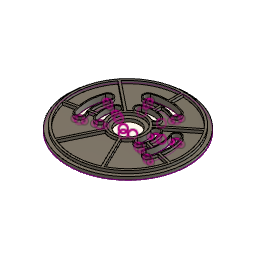
BoschRouterInsert (Autodesk Fusion 360 design; units mm, degrees)
Autodesk Fusion 360 part; units mm, degrees
sketch "Sketch1" plane through (0, 0, 0) normal (0, 1, 0) x (1, 0, 0)
  circle A0 centre (0, 0) radius 48.6
  circle A1 centre (0, 0) radius 9.35
  circle A2 centre (6.6396, 16.0293) radius 3
  circle A3 centre (-6.6396, 16.0293) radius 3
  arc A4 (7.7876, 18.8009) -> (-7.7876, 18.8009) centre (0, 0) ccw
  arc A5 (5.4915, 13.2577) -> (-5.4915, 13.2577) centre (0, 0) ccw
  line L0 (0, 55) -> (0, -55) construction
  circle A6 centre (-6.6396, 16.0293) radius 3.9
  circle A7 centre (6.6396, 16.0293) radius 3.9
  line L1 (0, 0) -> (25.3139, 61.1131) construction
  circle A8 centre (11.5379, 27.855) radius 3
  circle A9 centre (11.5379, 27.855) radius 3.9
  circle A10 centre (-11.5379, 27.855) radius 3
  circle A11 centre (-11.5379, 27.855) radius 3.9
  arc A12 (13.0304, 31.4581) -> (-13.0351, 31.4562) centre (0.0002, -3.0538) ccw
  arc A13 (10.0454, 24.2518) -> (-10.0454, 24.2518) centre (0, 0) ccw
  arc A14 (10.3899, 25.0833) -> (-10.3899, 25.0833) centre (0, 0) ccw
  arc A15 (12.686, 30.6266) -> (-12.6872, 30.6261) centre (0.0001, -3.8821) ccw
  arc A16 (8.132, 19.6324) -> (-8.132, 19.6324) centre (0, 0) ccw
  arc A17 (5.1471, 12.4262) -> (-5.1471, 12.4262) centre (0, 0) ccw
  dimension "d1" = 97.2
  dimension "d7" = 18.7
  dimension "d27" = 6
  dimension "d30" = 5
  dimension "d39" = 0.9
  dimension "d43" = 22.5
  dimension "d44" = 6
  dimension "d46" = 0.9
  dimension "d48" = 0.9
  dimension "d49" = 0.9
  dimension "d50" = 5
  constraint coincident A0.centre A1.centre
  constraint concentric A0 A1
  constraint coincident A3 A4.end
  constraint coincident A2 A4.start
  constraint coincident A3 A5.end
  constraint coincident A2 A5.start
  constraint tangent A2 A5
  constraint tangent A2 A4
  constraint tangent A3 A5
  constraint tangent A3 A4
  constraint vertical L0
  constraint symmetric A2 A3 L0
  constraint concentric A3 A6
  constraint concentric A2 A7
  constraint coincident A2.centre L1
  constraint coincident L1 A8.centre
  constraint concentric A8 A9
  constraint concentric A10 A11
  constraint symmetric L0 A8 A10
  constraint coincident A11 A12.end
  constraint coincident L1 A12.start
  constraint coincident A9 A12.start
  constraint coincident A11 A13.end
  constraint coincident L1 A13.start
  constraint coincident A9 A13.start
  constraint coincident A10 A14.end
  constraint coincident A8 A14.start
  constraint coincident L1 A14.start
  constraint coincident A10 A15.end
  constraint coincident A8 A15.start
  constraint coincident L1 A15.start
  constraint coincident A6 A16.end
  constraint coincident A7 A16.start
  constraint coincident L1 A16.start
  constraint coincident A6 A17.end
  constraint coincident L1 A17.start
  constraint coincident A7 A17.start
  measures "d1" diameter of A0
  measures "d7" diameter of A1
  measures "d27" diameter of A2
  measures "d30" distance of A1 A5
  measures "d39" distance of A3 A6
  measures "d43" angle of L0 L1
  measures "d44" diameter of A8
  measures "d46" distance of A8 A9
  measures "d48" distance of A10 A11
  measures "d49" distance of A2 A7
  measures "d50" distance of A13 A16
extrude "Extrude1" add sketch "Sketch1" along normal blind 2.5 contours A0 | A2 | A2 A4 A5 A7 | A2 A4 A5 A7 | A4 A5 A6 A7 | A4 A6 A7 A16 | A5 A6 A7 A17 | A3 A4 A5 A6 | A3 A4 A5 A6 | A3 | A8 A15 | A8 A9 A12 A14 A15 | A8 A15 | A8 A9 A14 A15 | A9 A11 A14 A15 | A9 A11 A13 A14 | A9 A11 A12 A15 | A10 A11 A14 A15 | A10 A11 A12 A14 A15 | A10 A15 | A10 A15
sketch "support_ribs" plane through (0, 2.5, 0) normal (0, 1, 0) x (-1, 0, 0)
  circle A0 centre (0, 0) radius 9.35
  circle A1 centre (0, 0) radius 48.6
  circle A2 centre (0, 0) radius 45.8
  circle A3 centre (0, 0) radius 44
  circle A4 centre (0, 0) radius 12.35
  circle A5 centre (0, 0) radius 14.15
  line L0 (-0.9352, -13.25) -> (0.8648, -13.25)
  line L1 (0.8648, -13.25) -> (0.8648, -44.9)
  line L2 (0.8648, -44.9) -> (-0.9352, -44.9)
  line L3 (-0.9352, -44.9) -> (-0.9352, -13.25)
  line L4 (-0.9352, -13.25) -> (0.8648, -44.9) construction
  line L5 (0.8648, -13.25) -> (-0.9352, -44.9) construction
  point P0 (-0.0352, -29.075)
  point P1 (-0.0352, -29.075)
  dimension "d12" = 91.6
  dimension "d13" = 88
  dimension "d14" = 24.7
  dimension "d15" = 28.3
  dimension "d16" = 29.075
  dimension "d17" = 1.8
  dimension "d18" = 31.65
  constraint coincident A0.centre A1.centre
  constraint concentric A2 A3
  constraint concentric A3 A4
  constraint perpendicular L0 L1
  constraint parallel L0 L2
  constraint parallel L1 L3
  constraint horizontal L0
  constraint coincident L4 P1
  constraint coincident L5 P1
  constraint coincident P1 P0
  measures "d12" diameter of A2
  measures "d13" diameter of A3
  measures "d14" diameter of A4
  measures "d15" diameter of A5
  measures "d16" vertical distance of A0.centre P1
  measures "d17" distance of L1.end L2.end
  measures "d18" distance of L0.end L1.end
extrude "Extrude2" add sketch "support_ribs" along normal blind 2.3 contours A2 | A3 L1 L2 L3 | A5 L0 L1 L3 | A5 L0 L1 L3
extrude "Extrude3" add sketch "support_ribs" along normal blind 2.3 contours A3 A5 L1 L3 picked at (-0.1352, -24.0974)
pattern_circular "C-Pattern1" count 7 over 360 about axis through (0, 1.75, 0) along (0, 1, 0) of "Extrude3"
extrude "Extrude5" add sketch "Sketch1" along normal blind 4.8 contours A2 A4 A5 A7 | A2 A4 A5 A7 | A4 A5 A6 A7 | A4 A6 A7 A16 | A5 A6 A7 A17 | A3 A4 A5 A6 | A3 A4 A5 A6 | A3 | A8 A9 A12 A14 A15 | A8 A9 A14 A15 | A9 A11 A14 A15 | A9 A11 A13 A14 | A9 A11 A12 A15 | A10 A11 A14 A15 | A10 A11 A12 A14 A15
extrude "Extrude4" cut sketch "Sketch1" along normal blind 14.8 contours A2 | A2 A4 A5 A7 | A4 A5 A6 A7 | A3 A4 A5 A6 | A3 | A8 A15 | A8 A15 | A8 A9 A14 A15 | A9 A11 A14 A15 | A10 A11 A14 A15 | A10 A15 | A10 A15 picked at (5.641, 19.3079) picked at (-5.6852, 19.3231)
chamfer "Chamfer1" distance 0.5 angle 45 4 edges at (0, 0, -14.35) (9.4112, 0, -14.8813) (0, 0, -20.35) (-9.4112, 0, -14.8813)
pattern_circular "C-Pattern2" count 3 over 180 about axis through (0, 1.75, 0) along (0, 1, 0) both ways of "Extrude5", "Extrude4", "Chamfer1"
sketch "Sketch3" plane through (0, 0, 0) normal (0, -1, 0) x (1, 0, 0)
  circle A0 centre (0, 0) radius 9.35
  arc A1 (-5.3002, -12.7957) -> (5.3002, -12.7957) centre (0, 0) ccw
  arc A2 (7.9789, -19.2629) -> (5.3002, -12.7957) centre (6.6396, -16.0293) ccw
  arc A3 (-7.9789, -19.2629) -> (7.9789, -19.2629) centre (0, 0) ccw
  arc A4 (-5.3002, -12.7957) -> (-7.9789, -19.2629) centre (-6.6396, -16.0293) ccw
  arc A5 (12.7957, -5.3002) -> (12.7957, 5.3002) centre (0, 0) ccw
  arc A6 (19.2629, 7.9789) -> (12.7957, 5.3002) centre (16.0293, 6.6396) ccw
  arc A7 (19.2629, -7.9789) -> (19.2629, 7.9789) centre (0, 0) ccw
  arc A8 (12.7957, -5.3002) -> (19.2629, -7.9789) centre (16.0293, -6.6396) ccw
  arc A9 (-12.7957, 5.3002) -> (-12.7957, -5.3002) centre (0, 0) ccw
  arc A10 (-19.2629, -7.9789) -> (-12.7957, -5.3002) centre (-16.0293, -6.6396) ccw
  arc A11 (-19.2629, 7.9789) -> (-19.2629, -7.9789) centre (0, 0) ccw
  arc A12 (-12.7957, 5.3002) -> (-19.2629, 7.9789) centre (-16.0293, 6.6396) ccw
  arc A13 (25.0833, -10.3899) -> (25.0833, 10.3899) centre (0, 0) ccw
  arc A14 (30.7168, 12.4379) -> (25.0833, 10.3899) centre (27.855, 11.5379) ccw
  arc A15 (30.7172, -12.4366) -> (30.7168, 12.4379) centre (-3.8821, 0.0001) ccw
  arc A16 (25.0833, -10.3899) -> (30.7172, -12.4366) centre (27.855, -11.5379) ccw
  arc A17 (-10.3899, -25.0833) -> (10.3899, -25.0833) centre (0, 0) ccw
  arc A18 (12.4379, -30.7168) -> (10.3899, -25.0833) centre (11.5379, -27.855) ccw
  arc A19 (-12.4366, -30.7172) -> (12.4379, -30.7168) centre (0.0001, 3.8821) ccw
  arc A20 (-10.3899, -25.0833) -> (-12.4366, -30.7172) centre (-11.5379, -27.855) ccw
  arc A21 (-25.0833, 10.3899) -> (-25.0833, -10.3899) centre (0, 0) ccw
  arc A22 (-30.7168, -12.4379) -> (-25.0833, -10.3899) centre (-27.855, -11.5379) ccw
  arc A23 (-30.7172, 12.4366) -> (-30.7168, -12.4379) centre (3.8821, -0.0001) ccw
  arc A24 (-25.0833, 10.3899) -> (-30.7172, 12.4366) centre (-27.855, 11.5379) ccw
  circle A25 centre (0, 0) radius 48.6
equation "d1 = insert_dia"
equation "insert_dia = 97.2 mm"
equation "bit_dia = 25.4 mm * 0.5"
equation "bit_clearance = 6 mm" comment "clearance between bit and insert"
equation "insert_thick = 2.5 mm"
equation "support_rib_height = 2.3 mm"
equation "d7 = bit_dia + bit_clearance"
equation "d8 = insert_thick"
equation "insert_lip = 2.8 mm"
equation "support_rib_width = 1.8 mm"
equation "d12 = insert_dia - 2 * insert_lip"
equation "d13 = insert_dia - 2 * insert_lip - support_rib_width * 2"
equation "d14 = bit_dia + 2 * bit_clearance"
equation "d15 = bit_dia + 2 * bit_clearance + 2 * support_rib_width"
equation "d16 = ( insert_dia - 2 * insert_lip - ( bit_dia + 2 * bit_clearance ) ) / 4 + bit_dia / 2 + bit_clearance"
equation "d17 = support_rib_width"
equation "d18 = insert_dia / 2 - insert_lip - bit_dia / 2 - bit_clearance - support_rib_width"
equation "d19 = support_rib_height"
equation "d21 = support_rib_height"
equation "d25 = insert_thick + support_rib_height + 10 mm"
equation "d27 = dusttrack_width"
equation "dusttrack_width = 6 mm" comment "opening width"
equation "d30 = dusttrack_spacing"
equation "d39 = support_rib_width * 0.5"
equation "d41 = support_rib_height + insert_thick"
equation "d44 = dusttrack_width"
equation "d46 = support_rib_width * 0.5"
equation "d48 = support_rib_width * 0.5"
equation "d49 = support_rib_width * 0.5"
equation "d50 = dusttrack_spacing"
equation "dusttrack_spacing = 5 mm"
